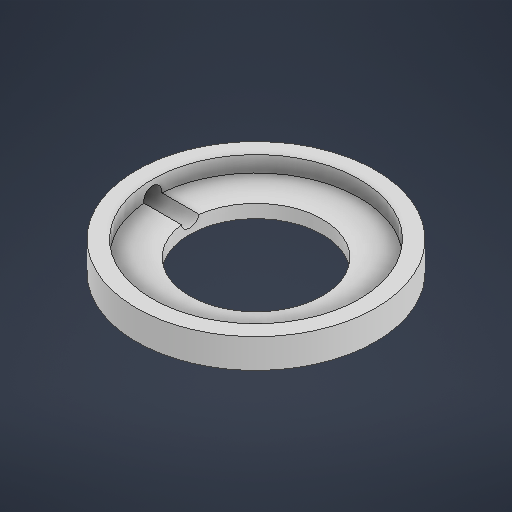
# Autodesk Inventor part: Part10
Saved by Autodesk Inventor 2025.2 (Build 292293000, 293)
## iProperties
Created: 2025-04-19
Part Number: Part10
Material: Generic
Document SubType Name: Modeling
Designer: klawy
Density: 1 g/cm^3
Appearance: Default
Author: klawy
Autodesk Inventor part; units mm, degrees
ref_plane "YZ Plane" through (0, 0, 0) normal (1, 0, 0) x (0, 1, 0)
ref_plane "XZ Plane" through (0, 0, 0) normal (0, 1, 0) x (-1, 0, 0)
ref_plane "XY Plane" through (0, 0, 0) normal (0, 0, 1) x (1, 0, 0)
sketch "Sketch1" plane through (0, 0, 0) normal (0, 0, 1) x (1, 0, 0)
  line L0 (22.5, 2.5) -> (12.5, 2.5)
  line L1 (12.5, 2.5) -> (12.5, 0)
  line L2 (12.5, 0) -> (22.5, 0)
  line L3 (22.5, 0) -> (22.5, 2.5)
  line L4 (22.5, 2.5) -> (12.5, 0) construction
  line L5 (12.5, 2.5) -> (22.5, 0) construction
  line L6 (22.5, 2.5) -> (19.5, 2.5)
  line L7 (19.5, 2.5) -> (19.5, 5.5)
  line L8 (19.5, 5.5) -> (22.5, 5.5)
  line L9 (22.5, 5.5) -> (22.5, 2.5)
  line L10 (0, -1.1) -> (0, 6.6) projected
  point P0 (0, 0)
  point P1 (17.5, 1.25)
  dimension "d0" = 12.5
  dimension "d1" = 10
  dimension "d2" = 2.5
  dimension "d3" = 3
  dimension "d4" = 3
  constraints: 20 end point, 4 parallel, 2 horizontal, 2 midpoint, 2 perpendicular, 1 point on line
  measures "d0" distance from line of point (0, 0) L1
  measures "d1" distance between parallel lines of L1 L3
  measures "d2" distance between parallel lines of L0 L2
  measures "d3" distance of L8.end L0.start
  measures "d4" distance of L7.end L8.end
revolve "Revolution1" add sketch "Sketch1" angle 360 about axis through (0, -10, 0) along (0, 1, 0)
sketch "Sketch2" plane through (0, 0, 0) normal (1, 0, 0) x (0, 1, 0)
  line L0 (0, 0) -> (5.5, 0)
  point P0 (2.75, 0)
  dimension "d6" = 5.5
  constraints: 2 end point, 1 horizontal, 1 midpoint
  measures "d6" distance of L0.start L0.end
hole "Hole1" at (0, 2.75, 0) direction (-1, 0, 0) diameter 3.4 end through all clearance for "Countersunk Flat Head Screw ISO 2009/7046" size "M3" standard "ISO"
body "Solid1"
